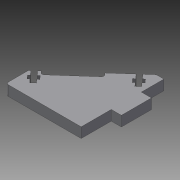
# Autodesk Inventor part: Mount_LCD_End_SD
Saved by Autodesk Inventor 2014 (Build 180170000, 170)
## iProperties
Created: 2014-10-26
Part Number: Mount_LCD_End_SD
Material: Generic
Document SubType Name: Modeling
Designer: ThatOtherGuy
Density: 1 g/cm^3
Appearance: Default
Author: ThatOtherGuy
Autodesk Inventor part; units mm, degrees
ref_plane "YZ Plane" through (0, 0, 0) normal (1, 0, 0) x (0, 1, 0)
ref_plane "XZ Plane" through (0, 0, 0) normal (0, 1, 0) x (-1, 0, 0)
ref_plane "XY Plane" through (0, 0, 0) normal (0, 0, 1) x (1, 0, 0)
sketch "Sketch1" plane through (0, 0, 0) normal (0, 0, 1) x (1, 0, 0)
  line L0 (0, 0) -> (50, 0)
  line L1 (50, 0) -> (50, 40)
  line L2 (50, 40) -> (56.731, 40)
  line L3 (56.731, 40) -> (56.731, 20)
  line L4 (56.731, 20) -> (50, 20)
  line L5 (50, 20) -> (50, 40)
  line L6 (10, 3.269) -> (30, 3.269)
  line L7 (30, 3.269) -> (30, 10)
  line L8 (30, 10) -> (10, 10)
  line L9 (10, 10) -> (10, 3.269)
  line L10 (0, 10) -> (10, 10)
  line L11 (30, 10) -> (50, 10)
  line L12 (0, 10) -> (0, 0)
  line L13 (0, 10) -> (0, 15)
  line L14 (0, 15) -> (45, 55)
  line L15 (50, 40) -> (50, 55)
  line L16 (50, 55) -> (45, 55)
  point P0 (20, 3.269)
  point P1 (20, 0)
  dimension "d2" = 20
  dimension "d3" = 20
  dimension "d5" = 6.731
  dimension "d6" = 10
  dimension "d9" = 10
  dimension "d11" = 20
  dimension "d12" = 20
  dimension "d14" = 5
  dimension "d16" = 15
  dimension "d17" = 5
  constraints: 34 end point, 7 perpendicular, 5 parallel, 3 horizontal, 2 collinear, 2 point on line, 1 coincident, 1 midpoint, 1 vertical alignment
  measures "d2" distance of L2.end L3.end
  measures "d3" distance of L7.end L8.end
  measures "d5" distance of L6.end L7.end
  measures "d6" distance between parallel lines of L0 L11
  measures "d9" distance between parallel lines of L9 L12
  measures "d11" distance between parallel lines of L1 L7
  measures "d12" distance between parallel lines of L0 L4
  measures "d14" distance of L10.start L13.end
  measures "d16" distance of L1.end L15.end
  measures "d17" distance of L15.end L14.end
extrude "Extrusion1" add sketch "Sketch1" along normal blind 6.731
sketch "Sketch2" plane through (0, 0, 6.731) normal (0, 0, 1) x (1, 0, 0)
  line L0 (45, 55) -> (0, 15) projected
  line L1 (4.4845, 18.9862) -> (6.5938, 16.6132)
  line L2 (6.5938, 16.6132) -> (29.0161, 36.5441)
  line L3 (29.0161, 36.5441) -> (26.9067, 38.9171)
  dimension "d18" = 3.175
  dimension "d19" = 30
  dimension "d20" = 6
  constraints: 6 end point, 3 perpendicular, 2 point on line
  measures "d18" distance between parallel lines of L0 L2
  measures "d19" distance of L1.end L2.end
  measures "d20" distance from line of L0.end L1
extrude "Extrusion2" cut sketch "Sketch2" against normal up to next
fillet "Fillet1" radius 1.5875 4 edges at (45, 55, 3.3655) (0, 0, 3.3655) (6.5938, 16.6132, 3.3655) (29.0161, 36.5441, 3.3655)
sketch "Sketch3" plane through (0, 0, 6.731) normal (0, 0, 1) x (1, 0, 0)
  line L0 (45, 55) -> (0, 15) projected
  line L1 (3.2333, 17.874) -> (5.7738, 15.0159)
  line L2 (5.7738, 15.0159) -> (6.8292, 15.954)
  line L3 (6.8292, 15.954) -> (8.9392, 13.5803)
  line L4 (8.9392, 13.5803) -> (7.8838, 12.6422)
  line L5 (7.8838, 12.6422) -> (9.8769, 10.3999)
  line L6 (9.8769, 10.3999) -> (7.5032, 8.2899)
  line L7 (7.5032, 8.2899) -> (5.5101, 10.5322)
  line L8 (5.5101, 10.5322) -> (4.4547, 9.5941)
  line L9 (4.4547, 9.5941) -> (2.3447, 11.9678)
  line L10 (2.3447, 11.9678) -> (3.4, 12.9059)
  line L11 (3.4, 12.9059) -> (0.8595, 15.764)
  line L12 (37.8802, 48.6713) -> (40.4207, 45.8132)
  line L13 (40.4207, 45.8132) -> (39.3654, 44.8751)
  line L14 (39.3654, 44.8751) -> (41.4754, 42.5013)
  line L15 (41.4754, 42.5013) -> (42.5307, 43.4394)
  line L16 (42.5307, 43.4394) -> (44.5238, 41.1972)
  line L17 (44.5238, 41.1972) -> (46.8976, 43.3072)
  line L18 (46.8976, 43.3072) -> (44.9045, 45.5494)
  line L19 (44.9045, 45.5494) -> (45.9598, 46.4875)
  line L20 (45.9598, 46.4875) -> (43.8498, 48.8613)
  line L21 (43.8498, 48.8613) -> (42.7945, 47.9232)
  line L22 (42.7945, 47.9232) -> (40.254, 50.7813)
  dimension "d24" = 3.176
  dimension "d25" = 10
  dimension "d26" = 3
  dimension "d27" = 6
  dimension "d28" = 1.15
  dimension "d29" = 6.35
  constraints: 44 end point, 13 parallel, 12 collinear, 8 equal length, 5 perpendicular, 4 point on line
  measures "d24" distance of L5.end L6.end
  measures "d25" distance between parallel lines of L0 L6
  measures "d26" distance between parallel lines of L6 L4
  measures "d27" distance between parallel lines of L9 L3
  measures "d28" distance from line of L0.end L11
  measures "d29" distance from line of L0.start L22
extrude "Extrusion3" cut sketch "Sketch3" against normal up to next
equation "\"d5\" = THICKB"
equation "\"d7\" = THICKB"
equation "\"THICKA\" = 3.175"
equation "\"THICKB\" = 6.731"
equation "\"THICKC\" = 12.7"
equation "\"THICKPLY\" = 5"
equation "\"MAGDIA\" = 9.5"
equation "\"BALLDIA\" = 12"
body "Solid1"
